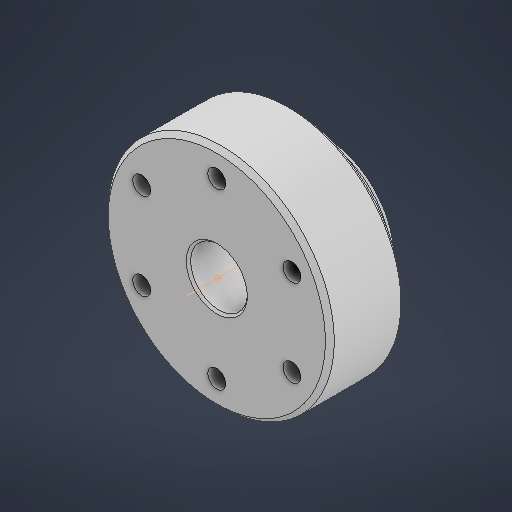
# Autodesk Inventor part: Porsche_912_CV_Joint
Saved by Autodesk Inventor 2027.1 (Build 311270010, 270A)
## iProperties
Created: 2026-08-06
Part Number: Porsche_912_CV_Joint
Material: Generic
Document SubType Name: Modeling
Designer: share
Density: 1 g/cm^3
Appearance: Default
Author: share
Autodesk Inventor part; units mm, degrees
ref_plane "YZ Plane" through (0, 0, 0) normal (1, 0, 0) x (0, 1, 0)
ref_plane "XZ Plane" through (0, 0, 0) normal (0, 1, 0) x (-1, 0, 0)
ref_plane "XY Plane" through (0, 0, 0) normal (0, 0, 1) x (1, 0, 0)
sketch "Sketch1" plane through (0, 0, 0) normal (0, 0, 1) x (1, 0, 0)
  circle A0 centre (0, 0) radius 12.7
  circle A1 centre (0, 0) radius 50.8
  dimension "d0" = 101.6
  dimension "d1" = 25.4
  constraints: 2 centre point, 2 coincident
  measures "d0" diameter of A1
  measures "d1" diameter of A0
extrude "Extrusion1" add sketch "Sketch1" along normal mid plane 34
sketch "Sketch2" plane through (0, 0, -17) normal (0, 0, -1) x (-1, 0, 0)
  circle A0 centre (0, 0) radius 39 construction
  circle A1 centre (0, 0) radius 12.7 construction
  line L0 (0, 0) -> (0, 39) construction
  dimension "d4" = 78
  constraints: 2 coincident, 2 end point, 1 vertical, 1 vertical alignment, 2 other
hole "Hole1" at (0, 39, -17) direction (0, 0, 1) diameter 8 end through all
pattern_circular "Circular Pattern1" count 6 over 360 about axis through (0, 0, -10) along (0, 0, 1) of "Hole1"
sketch "Sketch3" plane through (0, 0, -17) normal (0, 0, -1) x (-1, 0, 0)
  circle A0 centre (0, 0) radius 31.5
  circle A1 centre (0, 0) radius 12.7 projected
  dimension "d21" = 63
  constraints: 1 centre point, 1 coincident
  measures "d21" diameter of A0
extrude "Extrusion2" add sketch "Sketch3" along normal blind 15
fillet "Fillet1" radius 2 2 edges at (31.5, 0, -17) (31.5, 0, -32)
chamfer "Chamfer3" distance 2 angle 45 2 edges at (-50.8, 0, 17) (-50.8, 0, -17)
chamfer "Chamfer4" distance 1 angle 45 2 edges at (12.7, 0, -32) (-12.7, 0, 17)
body "Solid1"
